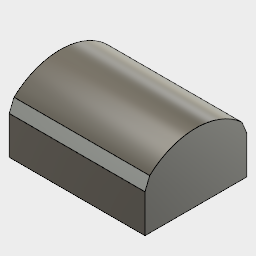
C05-W2-PE-02 (Autodesk Fusion 360 design; units mm, degrees)
Autodesk Fusion 360 part; units mm, degrees
sketch "Sketch1" plane through (0, 0, 0) normal (1, 0, 0) x (0, 0, -1)
  arc A0 (37.5, 33.0719) -> (-37.5, 33.0719) centre (0, 0) ccw
  line L0 (-37.5, 33.0719) -> (-37.5, 0)
  line L1 (-37.5, 0) -> (37.5, 0)
  line L2 (37.5, 0) -> (37.5, 33.0719)
  dimension "d1" = 50
  dimension "d2" = 75
  measures "d1" radius of A0
  measures "d2" distance of A0.start A0.end
extrude "Extrude1" add sketch "Sketch1" along normal mid plane 100
chamfer "Chamfer1" distance 5 angle 45 2 edges at (0, 33.0719, 37.5) (0, 33.0719, -37.5)
